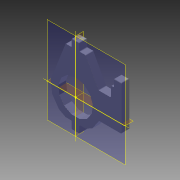
# Autodesk Inventor part: LenkungTeil1
Saved by Autodesk Inventor 2015 (Build 190159000, 159)
## iProperties
Created: 2018-10-20
Part Number: LenkungTeil1
Material: Generisch
Document SubType Name: Modeling
Designer: Boris
Density: 1 g/cm^3
Appearance: Vorgabe
Author: Boris
Autodesk Inventor part; units mm, degrees
sketch "Skizze1" plane through (0, 0, 0) normal (0, 1, 0) x (-1, 0, 0)
  line L0 (0, 11.3292) -> (5.2649, 10.0315)
  line L1 (5.2649, 10.0315) -> (9.3238, 6.4357)
  line L2 (9.3238, 6.4357) -> (11.2466, 1.3656)
  line L3 (11.2466, 1.3656) -> (10.593, -4.0174)
  line L4 (10.593, -4.0174) -> (7.5127, -8.48)
  line L5 (7.5127, -8.48) -> (2.7113, -11)
  line L6 (2.7113, -11) -> (-2.7113, -11)
  line L7 (-2.7113, -11) -> (-7.5127, -8.48)
  line L8 (-7.5127, -8.48) -> (-10.593, -4.0174)
  line L9 (-10.593, -4.0174) -> (-11.2466, 1.3656)
  line L10 (-11.2466, 1.3656) -> (-9.3238, 6.4357)
  line L11 (-9.3238, 6.4357) -> (-5.2649, 10.0315)
  line L12 (-5.2649, 10.0315) -> (0, 11.3292)
  line L13 (-6.5, 27) -> (-15, 11.3292)
  line L14 (-15.273, -5.7923) -> (-10.8318, -12.2265)
  line L15 (-10.8318, -12.2265) -> (-6.5, -14.5)
  line L16 (6.5, -14.5) -> (10.8318, -12.2265)
  line L17 (10.8318, -12.2265) -> (15.273, -5.7923)
  line L18 (15.273, -5.7923) -> (16.2154, 1.9689)
  line L19 (16.2154, 1.9689) -> (13.5619, 8.9656)
  line L20 (25.4584, 0) -> (-39.2431, 0) projected
  line L21 (2.5, 32) -> (-2.5, 32)
  line L22 (-2.5, 32) -> (-2.5, 27)
  line L23 (2.5, 27) -> (2.5, 32)
  line L24 (0, -29.8) -> (0, 42.3) projected
  line L25 (6.5, 27) -> (2.5, 27)
  line L26 (-2.5, 27) -> (-6.5, 27)
  line L27 (-2.5, -14.5) -> (-2.5, -19.5)
  line L28 (-2.5, -19.5) -> (2.5, -19.5)
  line L29 (2.5, -19.5) -> (2.5, -14.5)
  line L30 (-6.5, -14.5) -> (-2.5, -14.5)
  line L31 (2.5, -14.5) -> (6.5, -14.5)
  line L32 (-30, -5.721) -> (-15.2816, -5.721)
  line L33 (-25, 18) -> (-25, 23)
  line L34 (-15, 11.3292) -> (-23, 11.3292)
  line L35 (-23, 11.3292) -> (-23, 18)
  line L36 (-23, 18) -> (-25, 18)
  line L37 (-30, 23) -> (-30, -5.721)
  line L38 (-25, 23) -> (-30, 23)
  line L39 (6.5, 27) -> (13.5619, 8.9656)
  line L40 (-15.2816, -5.721) -> (-15.273, -5.7923)
  point P0 (0, 0)
  point P1 (0, 0)
  dimension "d42" = 28.721
  dimension "d43" = 32
  dimension "d44" = 19.5
  dimension "d45" = 8
  dimension "d46" = 30
  dimension "d47" = 5
  dimension "d48" = 4
  dimension "d49" = 4
  dimension "d50" = 4
  dimension "d51" = 4
  dimension "d52" = 5
  dimension "d53" = 15.8598
  dimension "d54" = 11
  dimension "d55" = 2
  dimension "d56" = 5
  dimension "d57" = 15.6708
  dimension "d58" = 11.3292
  dimension "d59" = 14.5
  dimension "d60" = 68.616
  dimension "d61" = 90
  dimension "d62" = 27
  dimension "d63" = 14.5
  dimension "d64" = 27
  dimension "d66" = 18
  constraints: 78 end point, 6 parallel, 5 horizontal, 3 perpendicular, 1 vertical, 33 other
  measures "d42" distance of L37.start L32.start
  measures "d43" distance between parallel lines of L20 L21
  measures "d44" distance between parallel lines of L20 L28
  measures "d45" distance of L13.end L34.end
  measures "d46" distance between parallel lines of L37 L24
  measures "d47" distance of L21.start L21.end
  measures "d48" distance of L22.end L13.start
  measures "d49" distance of L25.start L23.start
  measures "d50" distance of L29.end L16.start
  measures "d51" distance of L15.end L27.start
  measures "d52" distance of L27.end L28.end
  measures "d53" distance from line of point (0, 0) L18
  measures "d54" distance from line of point (0, 0) L3
  measures "d55" distance of L35.end L33.start
  measures "d56" distance of L33.end L37.start
  measures "d57" vertical distance of L13.start L13.end
  measures "d58" distance of point (0, 0) L0.start
  measures "d59" vertical distance of point (0, 0) L29.end
  measures "d60" angle of L39 L20
  measures "d61" angle of L31 L24
  measures "d62" distance between parallel lines of L25 L20
  measures "d63" distance between parallel lines of L30 L20
  measures "d64" distance between parallel lines of L26 L20
  measures "d66" distance between parallel lines of L36 L20
extrude "Extrusion1" add sketch "Skizze1" along normal blind 5 contours L24 L21 L23 L25 L39 L19 L18 L20 L3 L2 L1 L0 | L12 L11 L10 L9 L20 L37 L38 L33 L36 L35 L34 L13 L26 L22 L21 L24 | L20 L18 L17 L16 L31 L29 L28 L24 L6 L5 L4 L3 | L9 L8 L7 L6 L24 L28 L27 L30 L15 L14 L40 L32 L37 L20
fillet "Rundung1" radius 0.5 24 edges at (2.5, 2.5, 27) (6.5, 2.5, 27) (15, 2.5, 11.3292) (23, 2.5, 11.3292) (25, 2.5, 18) (23, 2.5, 18) (25, 2.5, 23) (27.5, 0, 23) (-2.5, 2.5, 27) (-6.5, 2.5, 27) (-2.5, 2.5, -14.5) (-2.5, 2.5, -19.5) (2.5, 2.5, -19.5) (2.5, 2.5, -14.5) (30, 2.5, -5.721) (15.273, 2.5, -5.7923) (30, 2.5, 23) (2.5, 2.5, 32) (-2.5, 2.5, 32) (27.5, 5, 23) (0, 5, 32) (0, 0, 32) (0, 0, -19.5) (0, 5, -19.5)
